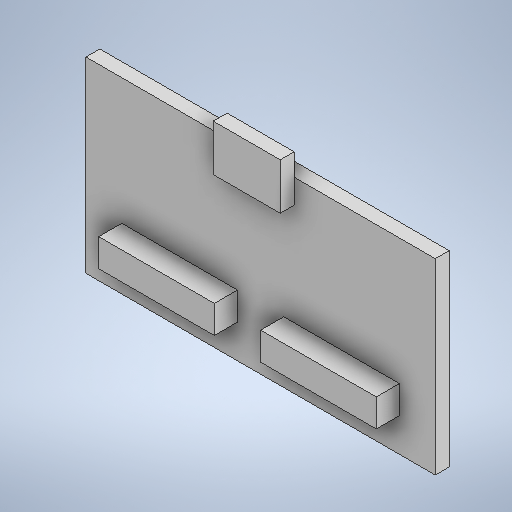
# Autodesk Inventor part: Pomodoro Robot Torso's back
Saved by Autodesk Inventor 2025.3 (Build 293356030, 356C)
## iProperties
Created: 2026-07-19
Part Number: Pomodoro Robot Torso's back
Material: Generic
Document SubType Name: Modeling
Designer: Samuel Correa Vega
Density: 1 g/cm^3
Appearance: Default
Author: Samuel Correa Vega
Autodesk Inventor part; units mm, degrees
ref_plane "YZ Plane" through (0, 0, 0) normal (1, 0, 0) x (0, 1, 0)
ref_plane "XY Plane" through (0, 0, 0) normal (0, 0, 1) x (1, 0, 0)
sketch "Sketch1" plane through (0, 0, 0) normal (0, 0, 1) x (1, 0, 0)
  line L0 (37.75, -20.25) -> (-37.75, -20.25)
  line L1 (-37.75, -20.25) -> (-37.75, 20.25)
  line L2 (-37.75, 20.25) -> (37.75, 20.25)
  line L3 (37.75, 20.25) -> (37.75, -20.25)
  point P0 (0, 0)
  point P1 (0, 20.25)
  point P2 (37.75, 0)
  dimension "d0" = 40.5
  dimension "d1" = 75.5
  constraints: 8 end point, 2 midpoint, 2 parallel, 1 horizontal, 1 horizontal alignment, 1 perpendicular, 1 vertical alignment
  measures "d0" distance of L0.end L1.end
  measures "d1" distance of L0.start L0.end
extrude "Extrusion1" add sketch "Sketch1" along normal blind 3
sketch "Sketch2" plane through (-37.75, 20.25, 0) normal (0, 1, 0) x (1, 0, 0)
  point P0 (37.75, 0)
ref_plane "Work Plane1" through (0, 15, 0) normal (0, 1, 0) x (-1, 0, 0)
sketch "Sketch3" plane through (0, 15, 0) normal (0, 1, 0) x (-1, 0, 0)
  line L0 (-37.75, 3) -> (37.75, 3) projected
  line L1 (7.25, 3) -> (-7.25, 3)
  line L2 (-7.25, 3) -> (-7.25, 6)
  line L3 (-7.25, 6) -> (7.25, 6)
  line L4 (7.25, 6) -> (7.25, 3)
  line L5 (7.25, 3) -> (-7.25, 3)
  point P0 (0, 6)
  point P1 (0, 3)
  dimension "d20" = 14.5
  dimension "d21" = 3
  constraints: 10 end point, 2 horizontal, 2 midpoint, 2 parallel, 1 perpendicular, 1 point on line, 1 vertical alignment
  measures "d20" distance of L2.end L3.end
  measures "d21" distance of L3.end L1.start
extrude "Extrusion2" add sketch "Sketch3" along normal blind 10
sketch "Sketch4" plane through (0, 0, 3) normal (0, 0, 1) x (1, 0, 0)
  line L0 (-30, -7) -> (-5, -7)
  line L1 (-5, -7) -> (-5, -13)
  line L2 (-5, -13) -> (-30, -13)
  line L3 (-30, -13) -> (-30, -7)
  line L4 (37.75, 20.25) -> (-37.75, 20.25) projected
  line L5 (0, 20.25) -> (0, -20.25) construction
  line L6 (-37.75, -20.25) -> (37.75, -20.25) projected
  line L7 (30, -7) -> (5, -7)
  line L8 (5, -7) -> (5, -13)
  line L9 (5, -13) -> (30, -13)
  line L10 (30, -13) -> (30, -7)
  point P0 (0, 0)
  point P1 (-5, -10)
  point P2 (-17.5, -7)
  point P3 (7.25, 20.25)
  point P4 (-7.25, 20.25)
  point P5 (0, 0)
  dimension "d9" = 25
  dimension "d10" = 6
  dimension "d11" = 5
  dimension "d12" = 7
  constraints: 18 end point, 5 midpoint, 4 symmetric about line, 2 parallel, 1 horizontal, 1 perpendicular
  measures "d9" distance of L1.end L2.end
  measures "d10" distance of L0.end L1.end
  measures "d11" distance from line of L1 point (0, 0)
  measures "d12" distance from line of L0 point (0, 0)
extrude "Extrusion3" add sketch "Sketch4" along normal blind 5
sketch "Sketch5" plane through (-30, -13, 3) normal (0, -1, 0) x (1, 0, 0)
  line L0 (25, 0) -> (0, 0) projected
  line L1 (5, 0) -> (20, 0)
  line L2 (20, 0) -> (20, 3.5)
  line L3 (20, 3.5) -> (5, 3.5)
  line L4 (5, 3.5) -> (5, 0)
  line L5 (35, 5) -> (60, 5) projected
  line L6 (0, 0) -> (0, 5) projected
  line L7 (0, 5) -> (25, 5) projected
  line L8 (30, -3) -> (30, 5) construction
  line L9 (55, 0) -> (40, 0)
  line L10 (40, 0) -> (40, 3.5)
  line L11 (40, 3.5) -> (55, 3.5)
  line L12 (55, 3.5) -> (55, 0)
  point P0 (47.5, 5)
  point P1 (0, 2.5)
  point P2 (12.5, 3.5)
  point P3 (12.5, 5)
  point P4 (47.5, 3.5)
  point P5 (20, 0)
  dimension "d15" = 15
  dimension "d16" = 3.5
  constraints: 18 end point, 5 symmetric about line, 4 midpoint, 2 parallel, 1 horizontal, 1 perpendicular, 1 point on line, 1 vertical, 1 vertical alignment
  measures "d15" distance of L2.end L3.end
  measures "d16" distance of L1.end L2.end
extrude "Extrusion4" cut sketch "Sketch5" against normal blind 3
body "Solid1"
